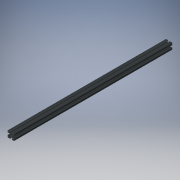
# Autodesk Inventor part: Профиль станочный 30x30x740
Saved by Autodesk Inventor 2019 (Build 230136000, 136)
## iProperties
Created: 2019-07-15
Part Number: Профиль станочный 30x30x740
Material: Чугун, литейный
Document SubType Name: Modeling
Designer: Петров Иван
Density: 7.15 g/cm^3
Appearance: Чугун серый
Author: Петров Иван
Autodesk Inventor part; units mm, degrees
ref_plane "YZ Plane" through (0, 0, 0) normal (1, 0, 0) x (0, 1, 0)
ref_plane "XZ Plane" through (0, 0, 0) normal (0, 1, 0) x (-1, 0, 0)
ref_plane "XY Plane" through (0, 0, 0) normal (0, 0, 1) x (1, 0, 0)
sketch "Эскиз1" plane through (0, 0, 0) normal (0, 0, 1) x (1, 0, 0)
  arc A0 (3.9646, 5.9999) -> (5.0253, 6.4392) centre (3.9646, 7.4999) ccw
  line L0 (3.9646, 5.9999) -> (0.7747, 5.9999)
  line L1 (0.7747, 5.9999) -> (0.0002, 5.35)
  line L2 (0.0002, 5.35) -> (-0.7746, 6.0001)
  line L3 (-0.7746, 6.0001) -> (-3.9642, 6.0001)
  arc A1 (-5.0249, 6.4394) -> (-3.9642, 6.0001) centre (-3.9642, 7.5001) ccw
  line L4 (-5.0249, 6.4394) -> (-8.3536, 9.7681)
  arc A2 (-8.5, 10.1217) -> (-8.3536, 9.7681) centre (-8, 10.1217) ccw
  line L5 (-8.5, 10.1217) -> (-8.5, 12.6)
  arc A3 (-8.3, 12.8) -> (-8.5, 12.6) centre (-8.3, 12.6) ccw
  line L6 (-8.3, 12.8) -> (-4.3, 12.8)
  arc A4 (-4.3, 12.8) -> (-4.1, 13) centre (-4.3, 13) ccw
  line L7 (-4.1, 13) -> (-4.1, 14.1)
  arc A5 (-4.1, 14.1) -> (-4.3, 14.3) centre (-4.3, 14.1) ccw
  line L8 (-4.3, 14.3) -> (-4.7, 14.3)
  line L9 (-4.7, 14.3) -> (-4.7, 14.8001)
  arc A6 (-4.7, 14.8001) -> (-4.9001, 15.0001) centre (-4.9001, 14.8001) ccw
  line L10 (-4.9001, 15.0001) -> (-13.5, 15.0001)
  arc A7 (-13.5, 15.0001) -> (-15, 13.5001) centre (-13.5, 13.5001) ccw
  line L11 (-15, 13.5001) -> (-15, 4.8999)
  arc A8 (-15, 4.8999) -> (-14.8, 4.6999) centre (-14.8, 4.8999) ccw
  line L12 (-14.8, 4.6999) -> (-14.3, 4.6999)
  line L13 (-14.3, 4.6999) -> (-14.3, 4.2999)
  arc A9 (-14.3, 4.2999) -> (-14.1, 4.0999) centre (-14.1, 4.2999) ccw
  line L14 (-14.1, 4.0999) -> (-13, 4.0999)
  arc A10 (-13, 4.0999) -> (-12.8, 4.2999) centre (-13, 4.2999) ccw
  line L15 (-12.8, 4.2999) -> (-12.8, 8.3)
  arc A11 (-12.6, 8.5) -> (-12.8, 8.3) centre (-12.6, 8.3) ccw
  line L16 (-12.6, 8.5) -> (-10.1211, 8.5)
  arc A12 (-9.7675, 8.3536) -> (-10.1211, 8.5) centre (-10.1211, 8) ccw
  line L17 (-9.7675, 8.3536) -> (-6.4392, 5.0253)
  arc A13 (-5.9999, 3.9646) -> (-6.4392, 5.0253) centre (-7.4999, 3.9646) ccw
  line L18 (-5.9999, 3.9646) -> (-5.9999, 0.7747)
  line L19 (-5.9999, 0.7747) -> (-5.35, 0.0002)
  line L20 (-5.35, 0.0002) -> (-6.0001, -0.7746)
  line L21 (-6.0001, -0.7746) -> (-6.0001, -3.9642)
  arc A14 (-6.4394, -5.0249) -> (-6.0001, -3.9642) centre (-7.5001, -3.9642) ccw
  line L22 (-6.4394, -5.0249) -> (-9.7681, -8.3536)
  arc A15 (-10.1217, -8.5) -> (-9.7681, -8.3536) centre (-10.1217, -8) ccw
  line L23 (-10.1217, -8.5) -> (-12.6, -8.5)
  arc A16 (-12.8, -8.3) -> (-12.6, -8.5) centre (-12.6, -8.3) ccw
  line L24 (-12.8, -8.3) -> (-12.8, -4.3)
  arc A17 (-12.8, -4.3) -> (-13, -4.1) centre (-13, -4.3) ccw
  line L25 (-13, -4.1) -> (-14.1, -4.1)
  arc A18 (-14.1, -4.1) -> (-14.3, -4.3) centre (-14.1, -4.3) ccw
  line L26 (-14.3, -4.3) -> (-14.3, -4.7)
  line L27 (-14.3, -4.7) -> (-14.8, -4.7)
  arc A19 (-14.8, -4.7) -> (-15, -4.9) centre (-14.8, -4.9) ccw
  line L28 (-15, -4.9) -> (-15, -13.5)
  arc A20 (-15, -13.5) -> (-13.5, -15) centre (-13.5, -13.5) ccw
  line L29 (-13.5, -15) -> (-4.8998, -15)
  arc A21 (-4.8998, -15) -> (-4.6998, -14.8) centre (-4.8998, -14.8) ccw
  line L30 (-4.6998, -14.8) -> (-4.6998, -14.3)
  line L31 (-4.6998, -14.3) -> (-4.2998, -14.3)
  arc A22 (-4.2998, -14.3) -> (-4.0998, -14.1) centre (-4.2998, -14.1) ccw
  line L32 (-4.0998, -14.1) -> (-4.0998, -13)
  arc A23 (-4.0998, -13) -> (-4.2998, -12.8) centre (-4.2998, -13) ccw
  line L33 (-4.2998, -12.8) -> (-8.2999, -12.8)
  arc A24 (-8.4999, -12.6) -> (-8.2999, -12.8) centre (-8.2999, -12.6) ccw
  line L34 (-8.4999, -12.6) -> (-8.4999, -10.1211)
  arc A25 (-8.3534, -9.7675) -> (-8.4999, -10.1211) centre (-7.9999, -10.1211) ccw
  line L35 (-8.3534, -9.7675) -> (-5.0251, -6.4392)
  arc A26 (-3.9645, -5.9999) -> (-5.0251, -6.4392) centre (-3.9645, -7.4999) ccw
  line L36 (-3.9645, -5.9999) -> (-0.7745, -5.9999)
  line L37 (-0.7745, -5.9999) -> (0, -5.35)
  line L38 (0, -5.35) -> (0.7747, -6.0001)
  line L39 (0.7747, -6.0001) -> (3.9644, -6.0001)
  arc A27 (5.025, -6.4394) -> (3.9644, -6.0001) centre (3.9644, -7.5001) ccw
  line L40 (5.025, -6.4394) -> (8.3537, -9.7681)
  arc A28 (8.5001, -10.1217) -> (8.3537, -9.7681) centre (8.0001, -10.1217) ccw
  line L41 (8.5001, -10.1217) -> (8.5001, -12.6)
  arc A29 (8.3001, -12.8) -> (8.5001, -12.6) centre (8.3001, -12.6) ccw
  line L42 (8.3001, -12.8) -> (4.3002, -12.8)
  arc A30 (4.3002, -12.8) -> (4.1002, -13) centre (4.3002, -13) ccw
  line L43 (4.1002, -13) -> (4.1002, -14.1)
  arc A31 (4.1002, -14.1) -> (4.3002, -14.3) centre (4.3002, -14.1) ccw
  line L44 (4.3002, -14.3) -> (4.7002, -14.3)
  line L45 (4.7002, -14.3) -> (4.7002, -14.8)
  arc A32 (4.7002, -14.8) -> (4.9002, -15) centre (4.9002, -14.8) ccw
  line L46 (4.9002, -15) -> (13.5001, -15)
  arc A33 (13.5001, -15) -> (15.0001, -13.5) centre (13.5001, -13.5) ccw
  line L47 (15.0001, -13.5) -> (15.0001, -4.8998)
  arc A34 (15.0001, -4.8998) -> (14.8001, -4.6998) centre (14.8001, -4.8998) ccw
  line L48 (14.8001, -4.6998) -> (14.3001, -4.6998)
  line L49 (14.3001, -4.6998) -> (14.3001, -4.2998)
  arc A35 (14.3001, -4.2998) -> (14.1001, -4.0998) centre (14.1001, -4.2998) ccw
  line L50 (14.1001, -4.0998) -> (13.0001, -4.0998)
  arc A36 (13.0001, -4.0998) -> (12.8001, -4.2998) centre (13.0001, -4.2998) ccw
  line L51 (12.8001, -4.2998) -> (12.8001, -8.2999)
  arc A37 (12.6001, -8.4999) -> (12.8001, -8.2999) centre (12.6001, -8.2999) ccw
  line L52 (12.6001, -8.4999) -> (10.1212, -8.4999)
  arc A38 (9.7677, -8.3534) -> (10.1212, -8.4999) centre (10.1212, -7.9999) ccw
  line L53 (9.7677, -8.3534) -> (6.4394, -5.0251)
  arc A39 (6, -3.9645) -> (6.4394, -5.0251) centre (7.5, -3.9645) ccw
  line L54 (6, -3.9645) -> (6, -0.7745)
  line L55 (6, -0.7745) -> (5.3501, 0)
  line L56 (5.3501, 0) -> (6.0002, 0.7747)
  line L57 (6.0002, 0.7747) -> (6.0002, 3.9644)
  arc A40 (6.4396, 5.025) -> (6.0002, 3.9644) centre (7.5002, 3.9644) ccw
  line L58 (6.4396, 5.025) -> (9.7682, 8.3537)
  arc A41 (10.1218, 8.5001) -> (9.7682, 8.3537) centre (10.1218, 8.0001) ccw
  line L59 (10.1218, 8.5001) -> (12.6001, 8.5001)
  arc A42 (12.8001, 8.3001) -> (12.6001, 8.5001) centre (12.6001, 8.3001) ccw
  line L60 (12.8001, 8.3001) -> (12.8001, 4.3002)
  arc A43 (12.8001, 4.3002) -> (13.0001, 4.1002) centre (13.0001, 4.3002) ccw
  line L61 (13.0001, 4.1002) -> (14.1001, 4.1002)
  arc A44 (14.1001, 4.1002) -> (14.3001, 4.3002) centre (14.1001, 4.3002) ccw
  line L62 (14.3001, 4.3002) -> (14.3001, 4.7001)
  line L63 (14.3001, 4.7001) -> (14.8001, 4.7001)
  arc A45 (14.8001, 4.7001) -> (15.0001, 4.9001) centre (14.8001, 4.9001) ccw
  line L64 (15.0001, 4.9001) -> (15.0001, 13.5002)
  arc A46 (15.0001, 13.5002) -> (13.5001, 15.0002) centre (13.5001, 13.5002) ccw
  line L65 (13.5001, 15.0002) -> (4.8999, 15.0002)
  arc A47 (4.8999, 15.0002) -> (4.6999, 14.8002) centre (4.8999, 14.8002) ccw
  line L66 (4.6999, 14.8002) -> (4.6999, 14.3)
  line L67 (4.6999, 14.3) -> (4.2999, 14.3)
  arc A48 (4.2999, 14.3) -> (4.0999, 14.1) centre (4.2999, 14.1) ccw
  line L68 (4.0999, 14.1) -> (4.0999, 13)
  arc A49 (4.0999, 13) -> (4.2999, 12.8) centre (4.2999, 13) ccw
  line L69 (4.2999, 12.8) -> (8.3, 12.8)
  arc A50 (8.5, 12.6) -> (8.3, 12.8) centre (8.3, 12.6) ccw
  line L70 (8.5, 12.6) -> (8.5, 10.1211)
  arc A51 (8.3536, 9.7675) -> (8.5, 10.1211) centre (8, 10.1211) ccw
  line L71 (8.3536, 9.7675) -> (5.0253, 6.4392)
  arc A52 (-12.7113, -10.2413) -> (-12.4546, -10.3134) centre (-12.5426, -10.1338) ccw
  arc A53 (-11.0457, -10.3134) -> (-12.4546, -10.3134) centre (-11.7501, -11.75) ccw
  arc A54 (-11.0457, -10.3134) -> (-10.789, -10.2413) centre (-10.9577, -10.1338) ccw
  line L72 (-10.6305, -9.9925) -> (-10.789, -10.2413)
  arc A55 (-10.4618, -9.9) -> (-10.6305, -9.9925) centre (-10.4618, -10.1) ccw
  line L73 (-10.3001, -9.9) -> (-10.4618, -9.9)
  arc A56 (-9.9001, -10.3) -> (-10.3001, -9.9) centre (-10.3001, -10.3) ccw
  line L74 (-9.9001, -10.4617) -> (-9.9001, -10.3)
  arc A57 (-9.9927, -10.6304) -> (-9.9001, -10.4617) centre (-10.1001, -10.4617) ccw
  line L75 (-10.2414, -10.7888) -> (-9.9927, -10.6304)
  arc A58 (-10.2414, -10.7888) -> (-10.3136, -11.0456) centre (-10.134, -10.9575) ccw
  arc A59 (-10.3136, -12.4544) -> (-10.3136, -11.0456) centre (-11.7501, -11.75) ccw
  arc A60 (-10.3136, -12.4544) -> (-10.2414, -12.7111) centre (-10.134, -12.5425) ccw
  line L76 (-9.9927, -12.8696) -> (-10.2414, -12.7111)
  arc A61 (-9.9001, -13.0383) -> (-9.9927, -12.8696) centre (-10.1001, -13.0383) ccw
  line L77 (-9.9001, -13.2) -> (-9.9001, -13.0383)
  arc A62 (-10.3001, -13.6) -> (-9.9001, -13.2) centre (-10.3001, -13.2) ccw
  line L78 (-10.4618, -13.6) -> (-10.3001, -13.6)
  arc A63 (-10.6305, -13.5075) -> (-10.4618, -13.6) centre (-10.4618, -13.4) ccw
  line L79 (-10.789, -13.2587) -> (-10.6305, -13.5075)
  arc A64 (-10.789, -13.2587) -> (-11.0457, -13.1866) centre (-10.9577, -13.3662) ccw
  arc A65 (-12.4546, -13.1866) -> (-11.0457, -13.1866) centre (-11.7501, -11.75) ccw
  arc A66 (-12.4546, -13.1866) -> (-12.7113, -13.2587) centre (-12.5426, -13.3662) ccw
  line L80 (-12.8698, -13.5075) -> (-12.7113, -13.2587)
  arc A67 (-13.0385, -13.6) -> (-12.8698, -13.5075) centre (-13.0385, -13.4) ccw
  line L81 (-13.2001, -13.6) -> (-13.0385, -13.6)
  arc A68 (-13.6001, -13.2) -> (-13.2001, -13.6) centre (-13.2001, -13.2) ccw
  line L82 (-13.6001, -13.0383) -> (-13.6001, -13.2)
  arc A69 (-13.5076, -12.8696) -> (-13.6001, -13.0383) centre (-13.4001, -13.0383) ccw
  line L83 (-13.2589, -12.7111) -> (-13.5076, -12.8696)
  arc A70 (-13.2589, -12.7111) -> (-13.1867, -12.4544) centre (-13.3663, -12.5425) ccw
  arc A71 (-13.1867, -11.0456) -> (-13.1867, -12.4544) centre (-11.7501, -11.75) ccw
  arc A72 (-13.1867, -11.0456) -> (-13.2589, -10.7888) centre (-13.3663, -10.9575) ccw
  line L84 (-13.5076, -10.6304) -> (-13.2589, -10.7888)
  arc A73 (-13.6001, -10.4617) -> (-13.5076, -10.6304) centre (-13.4001, -10.4617) ccw
  line L85 (-13.6001, -10.3) -> (-13.6001, -10.4617)
  arc A74 (-13.2001, -9.9) -> (-13.6001, -10.3) centre (-13.2001, -10.3) ccw
  line L86 (-13.0385, -9.9) -> (-13.2001, -9.9)
  arc A75 (-12.8698, -9.9925) -> (-13.0385, -9.9) centre (-13.0385, -10.1) ccw
  line L87 (-12.7113, -10.2413) -> (-12.8698, -9.9925)
  arc A76 (10.2413, -12.7113) -> (10.3134, -12.4546) centre (10.1338, -12.5426) ccw
  arc A77 (10.3134, -11.0457) -> (10.3134, -12.4546) centre (11.75, -11.7501) ccw
  arc A78 (10.3134, -11.0457) -> (10.2413, -10.789) centre (10.1338, -10.9577) ccw
  line L88 (9.9925, -10.6305) -> (10.2413, -10.789)
  arc A79 (9.9, -10.4618) -> (9.9925, -10.6305) centre (10.1, -10.4618) ccw
  line L89 (9.9, -10.3001) -> (9.9, -10.4618)
  arc A80 (10.3, -9.9001) -> (9.9, -10.3001) centre (10.3, -10.3001) ccw
  line L90 (10.4617, -9.9001) -> (10.3, -9.9001)
  arc A81 (10.6304, -9.9927) -> (10.4617, -9.9001) centre (10.4617, -10.1001) ccw
  line L91 (10.7888, -10.2414) -> (10.6304, -9.9927)
  arc A82 (10.7888, -10.2414) -> (11.0456, -10.3136) centre (10.9575, -10.134) ccw
  arc A83 (12.4544, -10.3136) -> (11.0456, -10.3136) centre (11.75, -11.7501) ccw
  arc A84 (12.4544, -10.3136) -> (12.7111, -10.2414) centre (12.5425, -10.134) ccw
  line L92 (12.8696, -9.9927) -> (12.7111, -10.2414)
  arc A85 (13.0383, -9.9001) -> (12.8696, -9.9927) centre (13.0383, -10.1001) ccw
  line L93 (13.2, -9.9001) -> (13.0383, -9.9001)
  arc A86 (13.6, -10.3001) -> (13.2, -9.9001) centre (13.2, -10.3001) ccw
  line L94 (13.6, -10.4618) -> (13.6, -10.3001)
  arc A87 (13.5075, -10.6305) -> (13.6, -10.4618) centre (13.4, -10.4618) ccw
  line L95 (13.2587, -10.789) -> (13.5075, -10.6305)
  arc A88 (13.2587, -10.789) -> (13.1866, -11.0457) centre (13.3662, -10.9577) ccw
  arc A89 (13.1866, -12.4546) -> (13.1866, -11.0457) centre (11.75, -11.7501) ccw
  arc A90 (13.1866, -12.4546) -> (13.2587, -12.7113) centre (13.3662, -12.5426) ccw
  line L96 (13.5075, -12.8698) -> (13.2587, -12.7113)
  arc A91 (13.6, -13.0385) -> (13.5075, -12.8698) centre (13.4, -13.0385) ccw
  line L97 (13.6, -13.2001) -> (13.6, -13.0385)
  arc A92 (13.2, -13.6001) -> (13.6, -13.2001) centre (13.2, -13.2001) ccw
  line L98 (13.0383, -13.6001) -> (13.2, -13.6001)
  arc A93 (12.8696, -13.5076) -> (13.0383, -13.6001) centre (13.0383, -13.4001) ccw
  line L99 (12.7111, -13.2589) -> (12.8696, -13.5076)
  arc A94 (12.7111, -13.2589) -> (12.4544, -13.1867) centre (12.5425, -13.3663) ccw
  arc A95 (11.0456, -13.1867) -> (12.4544, -13.1867) centre (11.75, -11.7501) ccw
  arc A96 (11.0456, -13.1867) -> (10.7888, -13.2589) centre (10.9575, -13.3663) ccw
  line L100 (10.6304, -13.5076) -> (10.7888, -13.2589)
  arc A97 (10.4617, -13.6001) -> (10.6304, -13.5076) centre (10.4617, -13.4001) ccw
  line L101 (10.3, -13.6001) -> (10.4617, -13.6001)
  arc A98 (9.9, -13.2001) -> (10.3, -13.6001) centre (10.3, -13.2001) ccw
  line L102 (9.9, -13.0385) -> (9.9, -13.2001)
  arc A99 (9.9925, -12.8698) -> (9.9, -13.0385) centre (10.1, -13.0385) ccw
  line L103 (10.2413, -12.7113) -> (9.9925, -12.8698)
  arc A100 (3.1213, -1.5836) -> (3.1996, -1.8473) centre (3.2996, -1.6741) ccw
  line L104 (3.7642, -2.1733) -> (3.1996, -1.8473)
  arc A101 (3.7642, -2.1733) -> (4.0056, -2.1415) centre (3.8642, -2.0001) ccw
  line L105 (4.1586, -1.9885) -> (4.0056, -2.1415)
  arc A102 (4.5, -2.13) -> (4.1586, -1.9885) centre (4.3, -2.13) ccw
  line L106 (4.5, -3.5) -> (4.5, -2.13)
  arc A103 (3.5, -4.5) -> (4.5, -3.5) centre (3.5, -3.5) ccw
  line L107 (2.13, -4.5) -> (3.5, -4.5)
  arc A104 (1.9885, -4.1586) -> (2.13, -4.5) centre (2.13, -4.3) ccw
  line L108 (2.1415, -4.0056) -> (1.9885, -4.1586)
  arc A105 (2.1415, -4.0056) -> (2.1733, -3.7642) centre (2.0001, -3.8642) ccw
  line L109 (1.8473, -3.1996) -> (2.1733, -3.7642)
  arc A106 (1.8473, -3.1996) -> (1.5836, -3.1213) centre (1.6741, -3.2996) ccw
  arc A107 (-1.5836, -3.1213) -> (1.5836, -3.1213) centre (0, 0) ccw
  arc A108 (-1.5836, -3.1213) -> (-1.8473, -3.1996) centre (-1.6741, -3.2996) ccw
  line L110 (-2.1733, -3.7642) -> (-1.8473, -3.1996)
  arc A109 (-2.1733, -3.7642) -> (-2.1415, -4.0056) centre (-2.0001, -3.8642) ccw
  line L111 (-1.9885, -4.1586) -> (-2.1415, -4.0056)
  arc A110 (-2.13, -4.5) -> (-1.9885, -4.1586) centre (-2.13, -4.3) ccw
  line L112 (-3.5, -4.5) -> (-2.13, -4.5)
  arc A111 (-4.5, -3.5) -> (-3.5, -4.5) centre (-3.5, -3.5) ccw
  line L113 (-4.5, -2.13) -> (-4.5, -3.5)
  arc A112 (-4.1586, -1.9885) -> (-4.5, -2.13) centre (-4.3, -2.13) ccw
  line L114 (-4.0056, -2.1415) -> (-4.1586, -1.9885)
  arc A113 (-4.0056, -2.1415) -> (-3.7642, -2.1733) centre (-3.8642, -2.0001) ccw
  line L115 (-3.1996, -1.8473) -> (-3.7642, -2.1733)
  arc A114 (-3.1996, -1.8473) -> (-3.1213, -1.5836) centre (-3.2996, -1.6741) ccw
  arc A115 (-3.1213, 1.5836) -> (-3.1213, -1.5836) centre (0, 0) ccw
  arc A116 (-3.1213, 1.5836) -> (-3.1996, 1.8473) centre (-3.2996, 1.6741) ccw
  line L116 (-3.7642, 2.1733) -> (-3.1996, 1.8473)
  arc A117 (-3.7642, 2.1733) -> (-4.0056, 2.1415) centre (-3.8642, 2.0001) ccw
  line L117 (-4.1586, 1.9885) -> (-4.0056, 2.1415)
  arc A118 (-4.5, 2.13) -> (-4.1586, 1.9885) centre (-4.3, 2.13) ccw
  line L118 (-4.5, 3.5) -> (-4.5, 2.13)
  arc A119 (-3.5, 4.5) -> (-4.5, 3.5) centre (-3.5, 3.5) ccw
  line L119 (-2.13, 4.5) -> (-3.5, 4.5)
  arc A120 (-1.9885, 4.1586) -> (-2.13, 4.5) centre (-2.13, 4.3) ccw
  line L120 (-2.1415, 4.0056) -> (-1.9885, 4.1586)
  arc A121 (-2.1415, 4.0056) -> (-2.1733, 3.7642) centre (-2.0001, 3.8642) ccw
  line L121 (-1.8473, 3.1996) -> (-2.1733, 3.7642)
  arc A122 (-1.8473, 3.1996) -> (-1.5836, 3.1213) centre (-1.6741, 3.2996) ccw
  arc A123 (1.5836, 3.1213) -> (-1.5836, 3.1213) centre (0, 0) ccw
  arc A124 (1.5836, 3.1213) -> (1.8473, 3.1996) centre (1.6741, 3.2996) ccw
  line L122 (2.1733, 3.7642) -> (1.8473, 3.1996)
  arc A125 (2.1733, 3.7642) -> (2.1415, 4.0056) centre (2.0001, 3.8642) ccw
  line L123 (1.9885, 4.1586) -> (2.1415, 4.0056)
  arc A126 (2.13, 4.5) -> (1.9885, 4.1586) centre (2.13, 4.3) ccw
  line L124 (3.5, 4.5) -> (2.13, 4.5)
  arc A127 (4.5, 3.5) -> (3.5, 4.5) centre (3.5, 3.5) ccw
  line L125 (4.5, 2.13) -> (4.5, 3.5)
  arc A128 (4.1586, 1.9885) -> (4.5, 2.13) centre (4.3, 2.13) ccw
  line L126 (4.0056, 2.1415) -> (4.1586, 1.9885)
  arc A129 (4.0056, 2.1415) -> (3.7642, 2.1733) centre (3.8642, 2.0001) ccw
  line L127 (3.1996, 1.8473) -> (3.7642, 2.1733)
  arc A130 (3.1996, 1.8473) -> (3.1213, 1.5836) centre (3.2996, 1.6741) ccw
  arc A131 (3.1213, -1.5836) -> (3.1213, 1.5836) centre (0, 0) ccw
  arc A132 (12.7113, 10.2413) -> (12.4546, 10.3134) centre (12.5426, 10.1338) ccw
  arc A133 (11.0457, 10.3134) -> (12.4546, 10.3134) centre (11.7501, 11.75) ccw
  arc A134 (11.0457, 10.3134) -> (10.789, 10.2413) centre (10.9577, 10.1338) ccw
  line L128 (10.6305, 9.9925) -> (10.789, 10.2413)
  arc A135 (10.4618, 9.9) -> (10.6305, 9.9925) centre (10.4618, 10.1) ccw
  line L129 (10.3001, 9.9) -> (10.4618, 9.9)
  arc A136 (9.9001, 10.3) -> (10.3001, 9.9) centre (10.3001, 10.3) ccw
  line L130 (9.9001, 10.4617) -> (9.9001, 10.3)
  arc A137 (9.9927, 10.6304) -> (9.9001, 10.4617) centre (10.1001, 10.4617) ccw
  line L131 (10.2414, 10.7888) -> (9.9927, 10.6304)
  arc A138 (10.2414, 10.7888) -> (10.3136, 11.0456) centre (10.134, 10.9575) ccw
  arc A139 (10.3136, 12.4544) -> (10.3136, 11.0456) centre (11.7501, 11.75) ccw
  arc A140 (10.3136, 12.4544) -> (10.2414, 12.7111) centre (10.134, 12.5425) ccw
  line L132 (9.9927, 12.8696) -> (10.2414, 12.7111)
  arc A141 (9.9001, 13.0383) -> (9.9927, 12.8696) centre (10.1001, 13.0383) ccw
  line L133 (9.9001, 13.2) -> (9.9001, 13.0383)
  arc A142 (10.3001, 13.6) -> (9.9001, 13.2) centre (10.3001, 13.2) ccw
  line L134 (10.4618, 13.6) -> (10.3001, 13.6)
  arc A143 (10.6305, 13.5075) -> (10.4618, 13.6) centre (10.4618, 13.4) ccw
  line L135 (10.789, 13.2587) -> (10.6305, 13.5075)
  arc A144 (10.789, 13.2587) -> (11.0457, 13.1866) centre (10.9577, 13.3662) ccw
  arc A145 (12.4546, 13.1866) -> (11.0457, 13.1866) centre (11.7501, 11.75) ccw
  arc A146 (12.4546, 13.1866) -> (12.7113, 13.2587) centre (12.5426, 13.3662) ccw
  line L136 (12.8698, 13.5075) -> (12.7113, 13.2587)
  arc A147 (13.0385, 13.6) -> (12.8698, 13.5075) centre (13.0385, 13.4) ccw
  line L137 (13.2001, 13.6) -> (13.0385, 13.6)
  arc A148 (13.6001, 13.2) -> (13.2001, 13.6) centre (13.2001, 13.2) ccw
  line L138 (13.6001, 13.0383) -> (13.6001, 13.2)
  arc A149 (13.5076, 12.8696) -> (13.6001, 13.0383) centre (13.4001, 13.0383) ccw
  line L139 (13.2589, 12.7111) -> (13.5076, 12.8696)
  arc A150 (13.2589, 12.7111) -> (13.1867, 12.4544) centre (13.3663, 12.5425) ccw
  arc A151 (13.1867, 11.0456) -> (13.1867, 12.4544) centre (11.7501, 11.75) ccw
  arc A152 (13.1867, 11.0456) -> (13.2589, 10.7888) centre (13.3663, 10.9575) ccw
  line L140 (13.5076, 10.6304) -> (13.2589, 10.7888)
  arc A153 (13.6001, 10.4617) -> (13.5076, 10.6304) centre (13.4001, 10.4617) ccw
  line L141 (13.6001, 10.3) -> (13.6001, 10.4617)
  arc A154 (13.2001, 9.9) -> (13.6001, 10.3) centre (13.2001, 10.3) ccw
  line L142 (13.0385, 9.9) -> (13.2001, 9.9)
  arc A155 (12.8698, 9.9925) -> (13.0385, 9.9) centre (13.0385, 10.1) ccw
  line L143 (12.7113, 10.2413) -> (12.8698, 9.9925)
  arc A156 (-10.2413, 12.7113) -> (-10.3134, 12.4546) centre (-10.1338, 12.5426) ccw
  arc A157 (-10.3134, 11.0457) -> (-10.3134, 12.4546) centre (-11.75, 11.7501) ccw
  arc A158 (-10.3134, 11.0457) -> (-10.2413, 10.789) centre (-10.1338, 10.9577) ccw
  line L144 (-9.9925, 10.6305) -> (-10.2413, 10.789)
  arc A159 (-9.9, 10.4618) -> (-9.9925, 10.6305) centre (-10.1, 10.4618) ccw
  line L145 (-9.9, 10.3001) -> (-9.9, 10.4618)
  arc A160 (-10.3, 9.9001) -> (-9.9, 10.3001) centre (-10.3, 10.3001) ccw
  line L146 (-10.4617, 9.9001) -> (-10.3, 9.9001)
  arc A161 (-10.6304, 9.9927) -> (-10.4617, 9.9001) centre (-10.4617, 10.1001) ccw
  line L147 (-10.7888, 10.2414) -> (-10.6304, 9.9927)
  arc A162 (-10.7888, 10.2414) -> (-11.0456, 10.3136) centre (-10.9575, 10.134) ccw
  arc A163 (-12.4544, 10.3136) -> (-11.0456, 10.3136) centre (-11.75, 11.7501) ccw
  arc A164 (-12.4544, 10.3136) -> (-12.7111, 10.2414) centre (-12.5425, 10.134) ccw
  line L148 (-12.8696, 9.9927) -> (-12.7111, 10.2414)
  arc A165 (-13.0383, 9.9001) -> (-12.8696, 9.9927) centre (-13.0383, 10.1001) ccw
  line L149 (-13.2, 9.9001) -> (-13.0383, 9.9001)
  arc A166 (-13.6, 10.3001) -> (-13.2, 9.9001) centre (-13.2, 10.3001) ccw
  line L150 (-13.6, 10.4618) -> (-13.6, 10.3001)
  arc A167 (-13.5075, 10.6305) -> (-13.6, 10.4618) centre (-13.4, 10.4618) ccw
  line L151 (-13.2587, 10.789) -> (-13.5075, 10.6305)
  arc A168 (-13.2587, 10.789) -> (-13.1866, 11.0457) centre (-13.3662, 10.9577) ccw
  arc A169 (-13.1866, 12.4546) -> (-13.1866, 11.0457) centre (-11.75, 11.7501) ccw
  arc A170 (-13.1866, 12.4546) -> (-13.2587, 12.7113) centre (-13.3662, 12.5426) ccw
  line L152 (-13.5075, 12.8698) -> (-13.2587, 12.7113)
  arc A171 (-13.6, 13.0385) -> (-13.5075, 12.8698) centre (-13.4, 13.0385) ccw
  line L153 (-13.6, 13.2001) -> (-13.6, 13.0385)
  arc A172 (-13.2, 13.6001) -> (-13.6, 13.2001) centre (-13.2, 13.2001) ccw
  line L154 (-13.0383, 13.6001) -> (-13.2, 13.6001)
  arc A173 (-12.8696, 13.5076) -> (-13.0383, 13.6001) centre (-13.0383, 13.4001) ccw
  line L155 (-12.7111, 13.2589) -> (-12.8696, 13.5076)
  arc A174 (-12.7111, 13.2589) -> (-12.4544, 13.1867) centre (-12.5425, 13.3663) ccw
  arc A175 (-11.0456, 13.1867) -> (-12.4544, 13.1867) centre (-11.75, 11.7501) ccw
  arc A176 (-11.0456, 13.1867) -> (-10.7888, 13.2589) centre (-10.9575, 13.3663) ccw
  line L156 (-10.6304, 13.5076) -> (-10.7888, 13.2589)
  arc A177 (-10.4617, 13.6001) -> (-10.6304, 13.5076) centre (-10.4617, 13.4001) ccw
  line L157 (-10.3, 13.6001) -> (-10.4617, 13.6001)
  arc A178 (-9.9, 13.2001) -> (-10.3, 13.6001) centre (-10.3, 13.2001) ccw
  line L158 (-9.9, 13.0385) -> (-9.9, 13.2001)
  arc A179 (-9.9925, 12.8698) -> (-9.9, 13.0385) centre (-10.1, 13.0385) ccw
  line L159 (-10.2413, 12.7113) -> (-9.9925, 12.8698)
  constraints: 360 point on circle, 320 end point, 180 centre point
extrude "Выдавливание1" add sketch "Эскиз1" against normal blind 740
